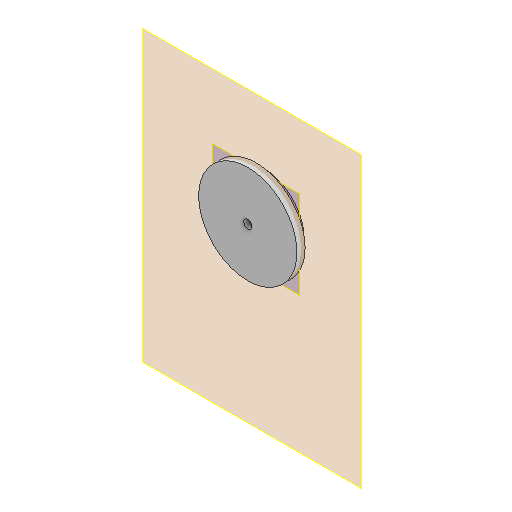
# Autodesk Inventor part: 20_Cube_Insert_Autofocus_KES400a_mirrorinsert_alignmenttube
Saved by Autodesk Inventor 2022 (Build 260153000, 153)
## iProperties
Created: 2023-06-16
Part Number: 20_Cube_Insert_Autofocus_KES400a_mirrorinsert_alignmenttube
Material: Generisch
Document SubType Name: Modeling
Designer: diederichbenedict
Density: 1 g/cm^3
Appearance: Vorgabe
Author: diederichbenedict
Autodesk Inventor part; units mm, degrees
ref_plane "YZ Plane" through (0, 0, 0) normal (1, 0, 0) x (0, 1, 0)
ref_plane "XZ Plane" through (0, 0, 0) normal (0, 1, 0) x (-1, 0, 0)
ref_plane "XY Plane" through (0, 0, 0) normal (0, 0, 1) x (1, 0, 0)
ref_plane "Arbeitsebene1" through (0, 0, 0) normal (0, 0, 1) x (1, 0, 0)
sketch "Skizze1" plane through (0, 0, 0) normal (0, 0, 1) x (1, 0, 0)
  line L0 (-6, -30.9) -> (-6, -18.4)
  line L1 (-6, -30.9) -> (-19.3, -30.9)
  line L2 (-19.3, -30.9) -> (-19.3, -33.9)
  line L3 (10.7, -33.9) -> (-19.3, -33.9)
  line L4 (10.7, -30.9) -> (10.7, -33.9)
  line L5 (10.7, -30.9) -> (6, -30.9)
  line L6 (6, -18.4) -> (6, -30.9)
  line L7 (16.5, -18.4) -> (6, -18.4)
  line L8 (16.5, -15.118081) -> (16.5, -18.4)
  line L9 (21.118081, -10.5) -> (16.5, -15.118081)
  line L10 (24.4, -10.5) -> (21.118081, -10.5)
  line L11 (24.4, 22.5) -> (24.4, -10.5)
  line L12 (21.118081, 22.5) -> (24.4, 22.5)
  line L13 (16.5, 27.118081) -> (21.118081, 22.5)
  line L14 (16.5, 30.4) -> (16.5, 27.118081)
  line L15 (-16.5, 30.4) -> (-2.249898, 30.4)
  line L16 (-16.5, 27.118081) -> (-16.5, 30.4)
  line L17 (-21.118081, 22.5) -> (-16.5, 27.118081)
  line L18 (-24.4, 22.5) -> (-21.118081, 22.5)
  line L19 (-24.4, -10.5) -> (-24.4, 22.5)
  line L20 (-21.118081, -10.5) -> (-24.4, -10.5)
  line L21 (-16.5, -15.118081) -> (-21.118081, -10.5)
  line L22 (-16.5, -18.4) -> (-16.5, -15.118081)
  line L23 (-6, -18.4) -> (-16.5, -18.4)
  spline S0 degree 2 poles (21.854355, -9.517776) (21.708528, -9.626528) (21.308123, -9.745166) (21.028828, -9.745166) knots 0 0 0 1 2 2 2
  spline S1 degree 2 poles (21.028828, -9.745166) (20.776721, -9.745166) (20.324412, -9.633942) (20.176113, -9.559793) knots 0 0 0 1 2 2 2
  line L24 (20.176113, -9.559793) -> (20.176113, -8.954242)
  line L25 (20.176113, -8.954242) -> (20.235433, -8.954242)
  spline S2 degree 2 poles (20.235433, -8.954242) (20.287337, -8.993788) (20.418334, -9.087711) (20.534501, -9.139615) knots 0 0 0 1 2 2 2
  spline S3 degree 2 poles (20.534501, -9.139615) (20.635838, -9.186576) (20.885473, -9.25331) (21.033771, -9.25331) knots 0 0 0 1 2 2 2
  spline S4 degree 2 poles (21.033771, -9.25331) (21.184541, -9.25331) (21.416875, -9.159388) (21.416875, -9.058051) knots 0 0 0 1 2 2 2
  spline S5 degree 2 poles (21.416875, -9.058051) (21.416875, -8.978959) (21.310595, -8.894923) (21.157353, -8.86032) knots 0 0 0 1 2 2 2
  spline S6 degree 2 poles (21.157353, -8.86032) (21.075789, -8.838075) (20.826154, -8.791114) (20.72976, -8.761455) knots 0 0 0 1 2 2 2
  spline S7 degree 2 poles (20.72976, -8.761455) (20.45788, -8.677419) (20.186, -8.348691) (20.186, -8.079283) knots 0 0 0 1 2 2 2
  spline S8 degree 2 poles (20.186, -8.079283) (20.186, -7.926041) (20.326883, -7.654161) (20.465295, -7.547881) knots 0 0 0 1 2 2 2
  spline S9 degree 2 poles (20.465295, -7.547881) (20.601235, -7.444072) (21.004112, -7.32049) (21.25869, -7.32049) knots 0 0 0 1 2 2 2
  spline S10 degree 2 poles (21.25869, -7.32049) (21.500911, -7.32049) (21.906259, -7.416884) (22.044671, -7.483618) knots 0 0 0 1 2 2 2
  line L26 (22.044671, -7.483618) -> (22.044671, -8.066925)
  line L27 (22.044671, -8.066925) -> (21.987823, -8.066925)
  spline S11 degree 2 poles (21.987823, -8.066925) (21.950749, -8.037265) (21.790092, -7.940871) (21.715943, -7.906268) knots 0 0 0 1 2 2 2
  spline S12 degree 2 poles (21.715943, -7.906268) (21.624493, -7.866722) (21.402045, -7.812346) (21.285878, -7.812346) knots 0 0 0 1 2 2 2
  spline S13 degree 2 poles (21.285878, -7.812346) (21.130165, -7.812346) (20.915133, -7.918626) (20.915133, -8.005134) knots 0 0 0 1 2 2 2
  spline S14 degree 2 poles (20.915133, -8.005134) (20.915133, -8.084226) (21.021413, -8.173205) (21.199371, -8.217694) knots 0 0 0 1 2 2 2
  spline S15 degree 2 poles (21.199371, -8.217694) (21.290822, -8.239939) (21.53057, -8.281957) (21.641794, -8.319032) knots 0 0 0 1 2 2 2
  spline S16 degree 2 poles (21.641794, -8.319032) (21.888958, -8.398124) (22.146008, -8.707079) (22.146008, -8.964129) knots 0 0 0 1 2 2 2
  spline S17 degree 2 poles (22.146008, -8.964129) (22.146008, -9.124785) (21.995238, -9.41891) (21.854355, -9.517776) knots 0 0 0 1 2 2 2
  spline S18 degree 2 poles (16.997588, -9.685847) (16.893779, -9.715506) (16.710878, -9.745166) (16.560108, -9.745166) knots 0 0 0 1 2 2 2
  spline S19 degree 2 poles (16.560108, -9.745166) (16.27587, -9.745166) (15.803787, -9.601811) (15.628301, -9.453513) knots 0 0 0 1 2 2 2
  spline S20 degree 2 poles (15.628301, -9.453513) (15.457758, -9.302743) (15.264971, -8.850434) (15.264971, -8.543951) knots 0 0 0 1 2 2 2
  spline S21 degree 2 poles (15.264971, -8.543951) (15.264971, -8.212751) (15.472588, -7.750555) (15.653018, -7.602257) knots 0 0 0 1 2 2 2
  spline S22 degree 2 poles (15.653018, -7.602257) (15.823561, -7.458902) (16.288228, -7.32049) (16.540335, -7.32049) knots 0 0 0 1 2 2 2
  spline S23 degree 2 poles (16.540335, -7.32049) (16.730651, -7.32049) (17.111283, -7.409469) (17.304071, -7.505863) knots 0 0 0 1 2 2 2
  line L28 (17.304071, -7.505863) -> (17.304071, -8.118829)
  line L29 (17.304071, -8.118829) -> (17.212621, -8.118829)
  spline S24 degree 2 poles (17.212621, -8.118829) (17.168131, -8.076811) (17.044549, -7.977946) (16.9704, -7.938399) knots 0 0 0 1 2 2 2
  spline S25 degree 2 poles (16.9704, -7.938399) (16.891308, -7.89391) (16.696048, -7.834591) (16.574938, -7.834591) knots 0 0 0 1 2 2 2
  spline S26 degree 2 poles (16.574938, -7.834591) (16.300587, -7.834591) (15.999047, -8.217694) (15.999047, -8.543951) knots 0 0 0 1 2 2 2
  spline S27 degree 2 poles (15.999047, -8.543951) (15.999047, -8.88998) (16.32036, -9.231066) (16.587296, -9.231066) knots 0 0 0 1 2 2 2
  spline S28 degree 2 poles (16.587296, -9.231066) (16.723236, -9.231066) (16.925911, -9.169275) (17.00006, -9.124785) knots 0 0 0 1 2 2 2
  spline S29 degree 2 poles (17.00006, -9.124785) (17.071737, -9.082767) (17.175546, -8.988845) (17.212621, -8.951771) knots 0 0 0 1 2 2 2
  line L30 (17.212621, -8.951771) -> (17.304071, -8.951771)
  line L31 (17.304071, -8.951771) -> (17.304071, -9.567208)
  spline S30 degree 2 poles (17.304071, -9.567208) (17.24228, -9.594396) (17.081624, -9.663602) (16.997588, -9.685847) knots 0 0 0 1 2 2 2
  spline S31 degree 2 poles (13.866024, -7.310604) (14.429557, -7.310604) (15.05241, -7.963116) (15.05241, -8.534064) knots 0 0 0 1 2 2 2
  spline S32 degree 2 poles (15.05241, -8.534064) (15.05241, -9.102541) (14.432029, -9.755053) (13.866024, -9.755053) knots 0 0 0 1 2 2 2
  spline S33 degree 2 poles (13.866024, -9.755053) (13.302491, -9.755053) (12.677167, -9.102541) (12.677167, -8.534064) knots 0 0 0 1 2 2 2
  spline S34 degree 2 poles (12.677167, -8.534064) (12.677167, -7.960644) (13.302491, -7.310604) (13.866024, -7.310604) knots 0 0 0 1 2 2 2
  spline S35 degree 2 poles (8.361688, -9.663602) (8.245522, -9.693262) (7.983528, -9.727865) (7.79074, -9.727865) knots 0 0 0 1 2 2 2
  spline S36 degree 2 poles (7.79074, -9.727865) (7.353261, -9.727865) (6.952855, -9.367006) (6.952855, -8.956714) knots 0 0 0 1 2 2 2
  line L32 (6.952855, -8.956714) -> (6.952855, -7.881552)
  line L33 (6.952855, -7.881552) -> (6.678504, -7.881552)
  line L34 (6.678504, -7.881552) -> (6.678504, -7.382281)
  line L35 (6.678504, -7.382281) -> (6.952855, -7.382281)
  line L36 (6.952855, -7.382281) -> (6.952855, -6.724826)
  line L37 (6.952855, -6.724826) -> (7.66963, -6.724826)
  line L38 (7.66963, -6.724826) -> (7.66963, -7.382281)
  line L39 (7.66963, -7.382281) -> (8.361688, -7.382281)
  line L40 (8.361688, -7.382281) -> (8.361688, -7.881552)
  line L41 (8.361688, -7.881552) -> (7.66963, -7.881552)
  line L42 (7.66963, -7.881552) -> (7.66963, -8.699664)
  spline S37 degree 2 poles (7.66963, -8.699664) (7.66963, -8.820774) (7.674573, -9.001203) (7.704233, -9.072881) knots 0 0 0 1 2 2 2
  spline S38 degree 2 poles (7.704233, -9.072881) (7.733893, -9.144558) (7.879719, -9.228594) (8.018131, -9.228594) knots 0 0 0 1 2 2 2
  spline S39 degree 2 poles (8.018131, -9.228594) (8.07745, -9.228594) (8.262823, -9.179161) (8.299898, -9.159388) knots 0 0 0 1 2 2 2
  line L43 (8.299898, -9.159388) -> (8.361688, -9.159388)
  line L44 (8.361688, -9.159388) -> (8.361688, -9.663602)
  spline S40 degree 2 poles (-8.240297, -8.729323) (-8.240297, -9.184105) (-8.9546, -9.737751) (-9.562623, -9.737751) knots 0 0 0 1 2 2 2
  spline S41 degree 2 poles (-9.562623, -9.737751) (-9.913596, -9.737751) (-10.442526, -9.601811) (-10.669917, -9.502946) knots 0 0 0 1 2 2 2
  line L45 (-10.669917, -9.502946) -> (-10.669917, -8.776284)
  line L46 (-10.669917, -8.776284) -> (-10.600711, -8.776284)
  spline S42 degree 2 poles (-10.600711, -8.776284) (-10.370848, -8.971544) (-9.819673, -9.181633) (-9.560152, -9.181633) knots 0 0 0 1 2 2 2
  spline S43 degree 2 poles (-9.560152, -9.181633) (-9.493417, -9.181633) (-9.278385, -9.151973) (-9.214122, -9.122314) knots 0 0 0 1 2 2 2
  spline S44 degree 2 poles (-9.214122, -9.122314) (-9.13503, -9.087711) (-9.023806, -8.961657) (-9.023806, -8.86032) knots 0 0 0 1 2 2 2
  spline S45 degree 2 poles (-9.023806, -8.86032) (-9.023806, -8.744153) (-9.204236, -8.600798) (-9.327818, -8.568667) knots 0 0 0 1 2 2 2
  spline S46 degree 2 poles (-9.327818, -8.568667) (-9.483531, -8.526649) (-9.836975, -8.454972) (-9.992688, -8.400596) knots 0 0 0 1 2 2 2
  spline S47 degree 2 poles (-9.992688, -8.400596) (-10.346132, -8.277014) (-10.652615, -7.854364) (-10.652615, -7.537994) knots 0 0 0 1 2 2 2
  spline S48 degree 2 poles (-10.652615, -7.537994) (-10.652615, -7.110401) (-9.928425, -6.578999) (-9.384665, -6.578999) knots 0 0 0 1 2 2 2
  spline S49 degree 2 poles (-9.384665, -6.578999) (-9.112785, -6.578999) (-8.573968, -6.690223) (-8.361408, -6.784145) knots 0 0 0 1 2 2 2
  line L47 (-8.361408, -6.784145) -> (-8.361408, -7.481147)
  line L48 (-8.361408, -7.481147) -> (-8.428142, -7.481147)
  spline S50 degree 2 poles (-8.428142, -7.481147) (-8.598685, -7.33532) (-9.088069, -7.135117) (-9.345119, -7.135117) knots 0 0 0 1 2 2 2
  spline S51 degree 2 poles (-9.345119, -7.135117) (-9.446456, -7.135117) (-9.604641, -7.164777) (-9.69362, -7.204323) knots 0 0 0 1 2 2 2
  spline S52 degree 2 poles (-9.69362, -7.204323) (-9.765297, -7.236455) (-9.869106, -7.36498) (-9.869106, -7.444072) knots 0 0 0 1 2 2 2
  spline S53 degree 2 poles (-9.869106, -7.444072) (-9.869106, -7.562711) (-9.703506, -7.698651) (-9.466229, -7.753027) knots 0 0 0 1 2 2 2
  spline S54 degree 2 poles (-9.466229, -7.753027) (-9.312988, -7.78763) (-9.02875, -7.854364) (-8.865622, -7.911211) knots 0 0 0 1 2 2 2
  spline S55 degree 2 poles (-8.865622, -7.911211) (-8.549252, -8.027378) (-8.240297, -8.412954) (-8.240297, -8.729323) knots 0 0 0 1 2 2 2
  line L49 (-14.466351, -8.049623) -> (-13.334341, -9.683375)
  line L50 (-13.334341, -9.683375) -> (-14.261205, -9.683375)
  line L51 (-14.261205, -9.683375) -> (-15.089204, -8.445085)
  line L52 (-15.089204, -8.445085) -> (-15.239973, -8.652703)
  line L53 (-15.239973, -8.652703) -> (-15.239973, -9.683375)
  line L54 (-15.239973, -9.683375) -> (-16.006181, -9.683375)
  line L55 (-16.006181, -9.683375) -> (-16.006181, -6.633375)
  line L56 (-16.006181, -6.633375) -> (-15.239973, -6.633375)
  line L57 (-15.239973, -6.633375) -> (-15.239973, -7.995247)
  line L58 (-15.239973, -7.995247) -> (-14.261205, -6.633375)
  line L59 (-14.261205, -6.633375) -> (-13.378831, -6.633375)
  line L60 (-13.378831, -6.633375) -> (-14.466351, -8.049623)
  line L61 (-11.023361, -9.683375) -> (-13.084706, -9.683375)
  line L62 (-13.084706, -9.683375) -> (-13.084706, -6.633375)
  line L63 (-13.084706, -6.633375) -> (-11.023361, -6.633375)
  line L64 (-11.023361, -6.633375) -> (-11.023361, -7.21421)
  line L65 (-11.023361, -7.21421) -> (-12.323442, -7.21421)
  line L66 (-12.323442, -7.21421) -> (-12.323442, -7.750555)
  line L67 (-12.323442, -7.750555) -> (-11.124698, -7.750555)
  line L68 (-11.124698, -7.750555) -> (-11.124698, -8.33139)
  line L69 (-11.124698, -8.33139) -> (-12.323442, -8.33139)
  line L70 (-12.323442, -8.33139) -> (-12.323442, -9.102541)
  line L71 (-12.323442, -9.102541) -> (-11.023361, -9.102541)
  line L72 (-11.023361, -9.102541) -> (-11.023361, -9.683375)
  line L73 (-5.575873, -8.42284) -> (-5.575873, -8.971544)
  line L74 (-5.575873, -8.971544) -> (-5.988636, -8.971544)
  line L75 (-5.988636, -8.971544) -> (-5.988636, -9.69079)
  line L76 (-5.988636, -9.69079) -> (-6.727655, -9.69079)
  line L77 (-6.727655, -9.69079) -> (-6.727655, -8.971544)
  line L78 (-6.727655, -8.971544) -> (-8.072226, -8.971544)
  line L79 (-8.072226, -8.971544) -> (-8.072226, -8.403067)
  line L80 (-8.072226, -8.403067) -> (-6.752372, -6.633375)
  line L81 (-6.752372, -6.633375) -> (-5.988636, -6.633375)
  line L82 (-5.988636, -6.633375) -> (-5.988636, -8.42284)
  line L83 (-5.988636, -8.42284) -> (-5.575873, -8.42284)
  spline S56 degree 2 poles (-3.245119, -6.984348) (-3.106707, -7.18455) (-2.980654, -7.775271) (-2.980654, -8.158375) knots 0 0 0 1 2 2 2
  spline S57 degree 2 poles (-2.980654, -8.158375) (-2.980654, -8.553837) (-3.106707, -9.14703) (-3.247591, -9.347233) knots 0 0 0 1 2 2 2
  spline S58 degree 2 poles (-3.247591, -9.347233) (-3.386002, -9.544964) (-3.833369, -9.747638) (-4.154681, -9.747638) knots 0 0 0 1 2 2 2
  spline S59 degree 2 poles (-4.154681, -9.747638) (-4.478466, -9.747638) (-4.92336, -9.544964) (-5.064244, -9.342289) knots 0 0 0 1 2 2 2
  spline S60 degree 2 poles (-5.064244, -9.342289) (-5.205127, -9.142087) (-5.331181, -8.553837) (-5.331181, -8.158375) knots 0 0 0 1 2 2 2
  spline S61 degree 2 poles (-5.331181, -8.158375) (-5.331181, -7.753027) (-5.205127, -7.179607) (-5.061772, -6.971989) knots 0 0 0 1 2 2 2
  spline S62 degree 2 poles (-5.061772, -6.971989) (-4.918417, -6.769315) (-4.466108, -6.571584) (-4.154681, -6.571584) knots 0 0 0 1 2 2 2
  spline S63 degree 2 poles (-4.154681, -6.571584) (-3.825954, -6.571584) (-3.386002, -6.779202) (-3.245119, -6.984348) knots 0 0 0 1 2 2 2
  spline S64 degree 2 poles (-0.573279, -6.984348) (-0.434868, -7.18455) (-0.308814, -7.775271) (-0.308814, -8.158375) knots 0 0 0 1 2 2 2
  spline S65 degree 2 poles (-0.308814, -8.158375) (-0.308814, -8.553837) (-0.434868, -9.14703) (-0.575751, -9.347233) knots 0 0 0 1 2 2 2
  spline S66 degree 2 poles (-0.575751, -9.347233) (-0.714163, -9.544964) (-1.161529, -9.747638) (-1.482842, -9.747638) knots 0 0 0 1 2 2 2
  spline S67 degree 2 poles (-1.482842, -9.747638) (-1.806626, -9.747638) (-2.251521, -9.544964) (-2.392404, -9.342289) knots 0 0 0 1 2 2 2
  spline S68 degree 2 poles (-2.392404, -9.342289) (-2.533287, -9.142087) (-2.659341, -8.553837) (-2.659341, -8.158375) knots 0 0 0 1 2 2 2
  spline S69 degree 2 poles (-2.659341, -8.158375) (-2.659341, -7.753027) (-2.533287, -7.179607) (-2.389933, -6.971989) knots 0 0 0 1 2 2 2
  spline S70 degree 2 poles (-2.389933, -6.971989) (-2.246578, -6.769315) (-1.794268, -6.571584) (-1.482842, -6.571584) knots 0 0 0 1 2 2 2
  spline S71 degree 2 poles (-1.482842, -6.571584) (-1.154114, -6.571584) (-0.714163, -6.779202) (-0.573279, -6.984348) knots 0 0 0 1 2 2 2
  line L84 (1.834095, -9.683375) -> (1.067888, -9.683375)
  line L85 (1.067888, -9.683375) -> (2.09856, -6.633375)
  line L86 (2.09856, -6.633375) -> (2.933974, -6.633375)
  line L87 (2.933974, -6.633375) -> (3.964646, -9.683375)
  line L88 (3.964646, -9.683375) -> (3.176194, -9.683375)
  line L89 (3.176194, -9.683375) -> (2.985878, -9.060523)
  line L90 (2.985878, -9.060523) -> (2.026883, -9.060523)
  line L91 (2.026883, -9.060523) -> (1.834095, -9.683375)
  line L92 (6.362134, -7.382281) -> (6.362134, -9.683375)
  line L93 (6.362134, -9.683375) -> (5.645359, -9.683375)
  line L94 (5.645359, -9.683375) -> (5.645359, -9.428797)
  spline S72 degree 2 poles (5.645359, -9.428797) (5.459987, -9.58451) (5.14856, -9.747638) (4.933528, -9.747638) knots 0 0 0 1 2 2 2
  spline S73 degree 2 poles (4.933528, -9.747638) (4.592442, -9.747638) (4.209338, -9.315101) (4.209338, -8.880093) knots 0 0 0 1 2 2 2
  line L95 (4.209338, -8.880093) -> (4.209338, -7.382281)
  line L96 (4.209338, -7.382281) -> (4.931056, -7.382281)
  line L97 (4.931056, -7.382281) -> (4.931056, -8.524177)
  spline S74 degree 2 poles (4.931056, -8.524177) (4.931056, -8.702135) (4.948358, -8.929526) (4.982961, -9.006147) knots 0 0 0 1 2 2 2
  spline S75 degree 2 poles (4.982961, -9.006147) (5.017564, -9.077824) (5.153504, -9.151973) (5.277085, -9.151973) knots 0 0 0 1 2 2 2
  spline S76 degree 2 poles (5.277085, -9.151973) (5.351235, -9.151973) (5.558852, -9.077824) (5.645359, -9.013562) knots 0 0 0 1 2 2 2
  line L98 (5.645359, -9.013562) -> (5.645359, -7.382281)
  line L99 (5.645359, -7.382281) -> (6.362134, -7.382281)
  spline S77 degree 2 poles (9.674128, -7.310604) (10.237661, -7.310604) (10.860513, -7.963116) (10.860513, -8.534064) knots 0 0 0 1 2 2 2
  spline S78 degree 2 poles (10.860513, -8.534064) (10.860513, -9.102541) (10.240133, -9.755053) (9.674128, -9.755053) knots 0 0 0 1 2 2 2
  spline S79 degree 2 poles (9.674128, -9.755053) (9.110594, -9.755053) (8.48527, -9.102541) (8.48527, -8.534064) knots 0 0 0 1 2 2 2
  spline S80 degree 2 poles (8.48527, -8.534064) (8.48527, -7.960644) (9.110594, -7.310604) (9.674128, -7.310604) knots 0 0 0 1 2 2 2
  line L100 (12.71177, -6.51968) -> (12.71177, -7.038724)
  line L101 (12.71177, -7.038724) -> (12.657394, -7.038724)
  spline S81 degree 2 poles (12.657394, -7.038724) (12.615376, -7.026365) (12.43989, -6.986819) (12.363269, -6.986819) knots 0 0 0 1 2 2 2
  spline S82 degree 2 poles (12.363269, -6.986819) (12.145765, -6.986819) (11.98758, -7.145004) (11.98758, -7.36498) knots 0 0 0 1 2 2 2
  line L102 (11.98758, -7.36498) -> (11.98758, -7.382281)
  line L103 (11.98758, -7.382281) -> (12.558528, -7.382281)
  line L104 (12.558528, -7.382281) -> (12.558528, -7.881552)
  line L105 (12.558528, -7.881552) -> (12.012296, -7.881552)
  line L106 (12.012296, -7.881552) -> (12.012296, -9.683375)
  line L107 (12.012296, -9.683375) -> (11.295522, -9.683375)
  line L108 (11.295522, -9.683375) -> (11.295522, -7.881552)
  line L109 (11.295522, -7.881552) -> (11.008812, -7.881552)
  line L110 (11.008812, -7.881552) -> (11.008812, -7.382281)
  line L111 (11.008812, -7.382281) -> (11.295522, -7.382281)
  line L112 (11.295522, -7.382281) -> (11.295522, -7.318019)
  spline S83 degree 2 poles (11.295522, -7.318019) (11.295522, -6.89784) (11.737945, -6.477662) (12.187783, -6.477662) knots 0 0 0 1 2 2 2
  spline S84 degree 2 poles (12.187783, -6.477662) (12.343496, -6.477662) (12.612904, -6.499907) (12.71177, -6.51968) knots 0 0 0 1 2 2 2
  line L113 (19.780651, -7.382281) -> (19.780651, -9.683375)
  line L114 (19.780651, -9.683375) -> (19.063877, -9.683375)
  line L115 (19.063877, -9.683375) -> (19.063877, -9.428797)
  spline S85 degree 2 poles (19.063877, -9.428797) (18.878504, -9.58451) (18.567078, -9.747638) (18.352045, -9.747638) knots 0 0 0 1 2 2 2
  spline S86 degree 2 poles (18.352045, -9.747638) (18.010959, -9.747638) (17.627856, -9.315101) (17.627856, -8.880093) knots 0 0 0 1 2 2 2
  line L116 (17.627856, -8.880093) -> (17.627856, -7.382281)
  line L117 (17.627856, -7.382281) -> (18.349574, -7.382281)
  line L118 (18.349574, -7.382281) -> (18.349574, -8.524177)
  spline S87 degree 2 poles (18.349574, -8.524177) (18.349574, -8.702135) (18.366875, -8.929526) (18.401478, -9.006147) knots 0 0 0 1 2 2 2
  spline S88 degree 2 poles (18.401478, -9.006147) (18.436081, -9.077824) (18.572021, -9.151973) (18.695603, -9.151973) knots 0 0 0 1 2 2 2
  spline S89 degree 2 poles (18.695603, -9.151973) (18.769752, -9.151973) (18.977369, -9.077824) (19.063877, -9.013562) knots 0 0 0 1 2 2 2
  line L119 (19.063877, -9.013562) -> (19.063877, -7.382281)
  line L120 (19.063877, -7.382281) -> (19.780651, -7.382281)
  arc A0 (2.5, 17.25833) -> (-11, 9.464102) centre (-2, 9.464102) ccw
  line L121 (8.5, 13.794229) -> (2.5, 17.25833)
  arc A1 (8.5, -1.794229) -> (8.5, 13.794229) centre (4, 6) ccw
  line L122 (2.5, -5.25833) -> (8.5, -1.794229)
  arc A2 (-11, 2.535898) -> (2.5, -5.25833) centre (-2, 2.535898) ccw
  line L123 (-11, 9.464102) -> (-11, 2.535898)
  line L124 (2, 16.392305) -> (8, 12.928203)
  line L125 (-10, 2.535898) -> (-10, 9.464102)
  line L126 (12, -3.206349) -> (-12, -3.206349)
  line L127 (8, -0.928203) -> (2, -4.392305)
  circle A3 centre (0, 6) radius 10
  circle A4 centre (0, 6) radius 1
  arc A5 (-2.249898, 30.4) -> (2.249898, 30.4) centre (0, 28.054695) ccw
  line L128 (2.249898, 30.4) -> (16.5, 30.4)
  point P0 (0, 0)
  dimension "d0" = 2
  constraints: 3 tangent, 2 centre point, 1 coincident
  measures "d0" diameter of A4
sketch "Skizze1 outline for Extrusion1" plane through (0, 0, 0) normal (0, 0, 1) x (1, 0, 0)
  circle A0 centre (0, 6) radius 10
  circle A1 centre (0, 6) radius 1
extrude "Extrusion1" add sketch "Skizze1 outline for Extrusion1" against normal blind 3 draft -5
ref_plane "Arbeitsebene2" through (0, 6, -1) normal (0, 0, -1) x (-1, 0, 0)
sketch "Skizze4" plane through (0, 6, -1) normal (0, 0, -1) x (-1, 0, 0)
  circle A0 centre (0, 0) radius 10
  circle A1 centre (0, 0) radius 9.737534
  point P0 (0, -6)
sketch "Skizze5" plane through (0, 6, 0) normal (0, 0, 1) x (1, 0, 0)
  circle A0 centre (0, 0) radius 1 projected
  circle A1 centre (0, 0) radius 10 projected
  circle A2 centre (0, 0) radius 1 projected
  circle A3 centre (0, 0) radius 12
  point P0 (0, -6)
  dimension "d9" = 24
  constraints: 1 centre point, 1 coincident
  measures "d9" diameter of A3
extrude "Extrusion4" add sketch "Skizze5" along normal mid plane 2 contours A1 | A3
